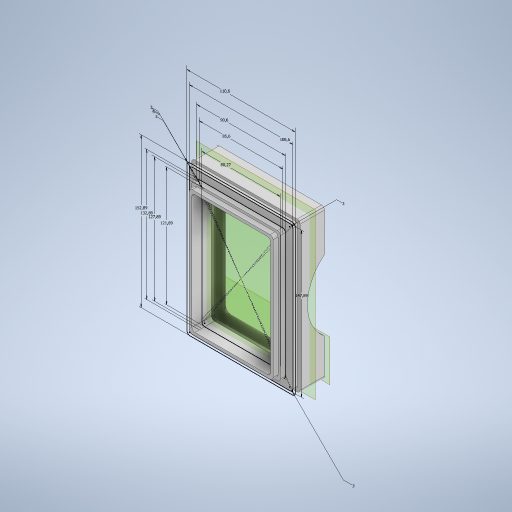
# Autodesk Inventor part: Halterung
Saved by Autodesk Inventor 2024 (Build 280153000, 153)
## iProperties
Created: 2024-02-26
Part Number: Halterung
Material: Generisch
Document SubType Name: Modeling
Designer: s1alknau
Density: 1 g/cm^3
Appearance: Vorgabe
Author: s1alknau
Autodesk Inventor part; units mm, degrees
ref_plane "YZ Plane" through (0, 0, 0) normal (1, 0, 0) x (0, 1, 0)
ref_plane "XZ Plane" through (0, 0, 0) normal (0, 1, 0) x (-1, 0, 0)
ref_plane "XY Plane" through (0, 0, 0) normal (0, 0, 1) x (1, 0, 0)
sketch "Skizze1" plane through (0, 0, 0) normal (0, 1, 0) x (-1, 0, 0)
  line L0 (-40.135, 57.945) -> (-40.135, -57.945)
  line L1 (-37.135, -60.945) -> (37.135, -60.945)
  line L2 (40.135, -57.945) -> (40.135, 57.945)
  line L3 (37.135, 60.945) -> (-37.135, 60.945)
  line L4 (-40.135, 60.945) -> (40.135, -60.945) construction
  line L5 (-40.135, -60.945) -> (40.135, 60.945) construction
  arc A0 (40.135, 57.945) -> (37.135, 60.945) centre (37.135, 57.945) ccw
  arc A1 (37.135, -60.945) -> (40.135, -57.945) centre (37.135, -57.945) ccw
  arc A2 (-40.135, -57.945) -> (-37.135, -60.945) centre (-37.135, -57.945) ccw
  arc A3 (-37.135, 60.945) -> (-40.135, 57.945) centre (-37.135, 57.945) ccw
  line L6 (-42.8, 60.945) -> (-42.8, -60.945)
  line L7 (-39.8, -63.945) -> (39.8, -63.945)
  line L8 (42.8, -60.945) -> (42.8, 60.945)
  line L9 (39.8, 63.945) -> (-39.8, 63.945)
  line L10 (-42.8, 63.945) -> (42.8, -63.945) construction
  line L11 (-42.8, -63.945) -> (42.8, 63.945) construction
  arc A4 (42.8, 60.945) -> (39.8, 63.945) centre (39.8, 60.945) ccw
  arc A5 (39.8, -63.945) -> (42.8, -60.945) centre (39.8, -60.945) ccw
  arc A6 (-42.8, -60.945) -> (-39.8, -63.945) centre (-39.8, -60.945) ccw
  arc A7 (-39.8, 63.945) -> (-42.8, 60.945) centre (-39.8, 60.945) ccw
  line L12 (-45.3, 63.445) -> (-45.3, -63.445)
  line L13 (-42.3, -66.445) -> (42.3, -66.445)
  line L14 (45.3, -63.445) -> (45.3, 63.445)
  line L15 (42.3, 66.445) -> (-42.3, 66.445)
  line L16 (-45.3, 66.445) -> (45.3, -66.445) construction
  line L17 (-45.3, -66.445) -> (45.3, 66.445) construction
  arc A8 (45.3, 63.445) -> (42.3, 66.445) centre (42.3, 63.445) ccw
  arc A9 (42.3, -66.445) -> (45.3, -63.445) centre (42.3, -63.445) ccw
  arc A10 (-45.3, -63.445) -> (-42.3, -66.445) centre (-42.3, -63.445) ccw
  arc A11 (-42.3, 66.445) -> (-45.3, 63.445) centre (-42.3, 63.445) ccw
  line L18 (-55.3, 73.445) -> (-55.3, -73.445)
  line L19 (-52.3, -76.445) -> (52.3, -76.445)
  line L20 (55.3, -73.445) -> (55.3, 73.445)
  line L21 (52.3, 76.445) -> (-52.3, 76.445)
  line L22 (-55.3, 76.445) -> (55.3, -76.445) construction
  line L23 (-55.3, -76.445) -> (55.3, 76.445) construction
  arc A12 (55.3, 73.445) -> (52.3, 76.445) centre (52.3, 73.445) ccw
  arc A13 (52.3, -76.445) -> (55.3, -73.445) centre (52.3, -73.445) ccw
  arc A14 (-55.3, -73.445) -> (-52.3, -76.445) centre (-52.3, -73.445) ccw
  arc A15 (-52.3, 76.445) -> (-55.3, 73.445) centre (-52.3, 73.445) ccw
  line L24 (52.8, -70.945) -> (52.8, 70.945)
  line L25 (49.8, 73.945) -> (-49.8, 73.945)
  line L26 (-52.8, 70.945) -> (-52.8, -70.945)
  line L27 (-49.8, -73.945) -> (49.8, -73.945)
  line L28 (52.8, -73.945) -> (-52.8, 73.945) construction
  line L29 (52.8, 73.945) -> (-52.8, -73.945) construction
  arc A16 (-52.8, -70.945) -> (-49.8, -73.945) centre (-49.8, -70.945) ccw
  arc A17 (-49.8, 73.945) -> (-52.8, 70.945) centre (-49.8, 70.945) ccw
  arc A18 (52.8, 70.945) -> (49.8, 73.945) centre (49.8, 70.945) ccw
  arc A19 (49.8, -73.945) -> (52.8, -70.945) centre (49.8, -70.945) ccw
  point P0 (0, 0)
  dimension "d0" = 121.89
  dimension "d1" = 80.27
  dimension "d2" = 3
  dimension "d3" = 127.89
  dimension "d4" = 85.6
  dimension "d5" = 3
  dimension "d6" = 3
  dimension "d7" = 90.6
  dimension "d8" = 132.89
  dimension "d9" = 3
  dimension "d10" = 152.89
  dimension "d11" = 110.6
  dimension "d20" = 147.89
  dimension "d21" = 105.6
  dimension "d22" = 3
  dimension "d23" = 3
  constraints: 60 end point, 40 point on circle, 40 point on line, 40 tangent, 20 centre point, 14 equal radius, 10 midpoint, 10 parallel, 5 perpendicular, 5 vertical
  measures "d0" distance between parallel lines of L1 L3
  measures "d1" distance between parallel lines of L2 L0
  measures "d2" radius of A0
  measures "d3" distance between parallel lines of L7 L9
  measures "d4" distance between parallel lines of L8 L6
  measures "d5" radius of A4
  measures "d6" radius of A8
  measures "d7" distance between parallel lines of L14 L12
  measures "d8" distance between parallel lines of L13 L15
  measures "d9" radius of A12
  measures "d10" distance between parallel lines of L19 L21
  measures "d11" distance between parallel lines of L20 L18
  measures "d20" distance between parallel lines of L25 L27
  measures "d21" distance between parallel lines of L26 L24
  measures "d22" radius of A16
  measures "d23" radius of A17
extrude "Extrusion1" add sketch "Skizze1" along normal blind 10 and the other way blind 10 contours A7 L9 A4 L8 A5 L7 A6 L6
extrude "Extrusion2" add sketch "Skizze1" along normal blind 10 and the other way blind 5 contours A11 L15 A8 L14 A9 L13 A10 L12
ref_plane "Arbeitsebene1" through (0, 5, 0) normal (0, 1, 0) x (1, 0, 0)
extrude "Extrusion5" add sketch "Skizze1" along normal blind 5 and the other way blind 5 from surface at 5 contours A19 L27 A16 L26 A17 L25 A18 L24
extrude "Extrusion6" add sketch "Skizze1" along normal blind 25 from surface at 5 contours A15 L21 A12 L20 A13 L19 A14 L18
extrude "Extrusion7" add sketch "Skizze1" against normal blind 4 from surface at 30 contours A7 L9 A4 L8 A5 L7 A6 L6 | A11 L15 A8 L14 A9 L13 A10 L12 | A19 L27 A16 L26 A17 L25 A18 L24
sketch "Skizze2" plane through (55.3, 5, 73.445) normal (1, 0, 0) x (0, 0, -1)
  line L0 (146.89, 25) -> (0, 25) projected
  arc A0 (39.3256, 25) -> (111.3463, 25) centre (75.336, 53.4449) ccw
  point P0 (73.445, -5)
  constraints: 2 point on circle, 2 point on line, 1 centre point
extrude "Extrusion8" cut sketch "Skizze2" against normal blind 16.25
ref_plane "Arbeitsebene2" through (0, 15, 0) normal (0, 1, 0) x (-1, 0, 0)
ref_plane "Arbeitsebene3" through (-52.3, 30, -76.445) normal (0, 1, 0) x (1, 0, 0)
extrude "Extrusion9" cut sketch "Skizze1" against normal blind 5 from surface at 30 contours A3 L3 A0 L2 A1 L1 A2 L0 | A7 L9 A4 L8 A5 L7 A6 L6
chamfer "Fasen3" distance 3 angle 45 9 edges at (0, 30, 63.945) (-41.9213, 30, 63.0663) (-42.8, 30, 0) (41.9213, 30, 63.0663) (42.8, 30, 47.5322) (-41.9213, 30, -63.0663) (0, 30, -63.945) (41.9213, 30, -63.0663) (42.8, 30, -49.4231)
